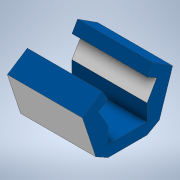
# Autodesk Inventor part: защёлка_выдача
Saved by Autodesk Inventor 2020 (Build 240168000, 168)
## iProperties
Created: 2022-07-29
Part Number: защёлка_выдача
Material: Типовые
Document SubType Name: Modeling
Designer: akapu
Density: 1 g/cm^3
Appearance: По умолчанию
Author: akapu
Autodesk Inventor part; units mm, degrees
ref_plane "YZ Plane" through (0, 0, 0) normal (1, 0, 0) x (0, 1, 0)
ref_plane "XZ Plane" through (0, 0, 0) normal (0, 1, 0) x (-1, 0, 0)
ref_plane "XY Plane" through (0, 0, 0) normal (0, 0, 1) x (1, 0, 0)
sketch "Эскиз8" plane through (0, 0, 0) normal (1, 0, 0) x (0, 1, 0)
  line L0 (0, 0) -> (10.4, 0)
  line L1 (10.4, 0) -> (10.4, -10.4)
  line L2 (10.4, -10.4) -> (0, -10.4)
  line L3 (0, -10.4) -> (0, 0)
  line L4 (5.2, 0) -> (5.2, 4)
  line L5 (5.2, -10.4) -> (5.2, -14.4)
  circle A0 centre (5.2, 4) radius 1.6
  circle A1 centre (5.2, -14.4) radius 1.6
  line L6 (5.2, 4) -> (7.9, 4)
  line L7 (7.9, 2.4412) -> (5.2, 0.8823)
  line L8 (5.2, 0.8823) -> (2.5, 2.4412)
  line L9 (2.5, 2.4412) -> (2.5, 5.5588)
  line L10 (2.5, 5.5588) -> (5.2, 7.1177)
  line L11 (5.2, 7.1177) -> (7.9, 5.5588)
  line L12 (7.9, 5.5588) -> (7.9, 2.4412)
  line L13 (7.9, -15.9588) -> (5.2, -17.5177)
  line L14 (5.2, -17.5177) -> (2.5, -15.9588)
  line L15 (2.5, -15.9588) -> (2.5, -12.8412)
  line L16 (2.5, -12.8412) -> (5.2, -11.2823)
  line L17 (5.2, -11.2823) -> (7.9, -12.8412)
  line L18 (7.9, -12.8412) -> (7.9, -15.9588)
  circle A2 centre (5.2, 4) radius 5.2
  circle A3 centre (5.2, -14.4) radius 5.2
  line L19 (10.4, 4) -> (10.4, 0)
  line L20 (10.4, -10.4) -> (10.4, -14.4)
  line L21 (0, -14.4) -> (0, -10.4)
  line L22 (0, 4) -> (0, 0)
  line L23 (7.9, 5.5588) -> (7.9, 8.4441)
  line L24 (2.5, 5.5588) -> (2.5, 8.4441)
  line L25 (2.5, -15.9588) -> (2.5, -18.8441)
  line L26 (7.9, -15.9588) -> (7.9, -18.8441)
  line L27 (0, 0) -> (-3, 0)
  line L28 (-3, 0) -> (-3, -10.4)
  line L29 (-3, -10.4) -> (0, -10.4)
  line L30 (0, -10.4) -> (0, 0)
  line L31 (10.4, 0) -> (8.9, 2.5981)
  line L32 (10.4, -10.4) -> (8.9, -12.9981)
  line L33 (10.4, -10.4) -> (13.4, -10.4) construction
  line L34 (8.9, -12.9981) -> (4.4, -10.4)
  line L35 (8.9, 2.5981) -> (4.4, 0)
  line L36 (-3, 0) -> (0.663, 6.5408)
  line L37 (-3, -10.4) -> (0.663, -16.9408)
  line L38 (10.4, 0) -> (12.9981, 1.5)
  line L39 (12.9981, 1.5) -> (9.5707, 6.8173)
  line L40 (10.4, -10.4) -> (12.9981, -11.9)
  line L41 (12.9981, -11.9) -> (9.5707, -17.2173)
  point P0 (7.9, -14.4)
  dimension "d51" = 10.4
  dimension "d52" = 10.4
  dimension "d53" = 4
  dimension "d54" = 4
  dimension "d55" = 3.2
  dimension "d56" = 3.2
  dimension "d57" = 2.7
  dimension "d58" = 3
  dimension "d59" = 3
  dimension "d60" = 3
  dimension "d61" = 120
  dimension "d62" = 3
  dimension "d63" = 3
  constraints: 84 end point, 12 point on circle, 7 tangent, 6 coincident, 6 parallel, 6 point on line, 5 perpendicular, 4 centre point, 4 midpoint, 4 vertical, 3 horizontal, 1 collinear, 1 equal length, 26 other
  measures "d51" distance of L1.end L2.end
  measures "d52" distance of L0.end L1.end
  measures "d53" distance of L4.start L4.end
  measures "d54" distance of L5.start L5.end
  measures "d55" diameter of A0
  measures "d56" diameter of A1
  measures "d57" distance of L6.start L6.end
  measures "d58" distance of L29.end L28.end
  measures "d59" distance of L0.end L31.end
  measures "d60" distance of L1.end L32.end
  measures "d61" angle of L32 L33
  measures "d62" distance of L0.end L38.end
  measures "d63" distance of L1.end L40.end
extrude "Выдавливание6" add sketch "Эскиз8" along normal blind 5 contours L0 A2 L24 L9 L8 L4 L35 | L0 L22 A2 | L4 L7 L12 L23 A2 L31 L35 | L27 L36 A2 L22 | L3 L29 L28 L27 | L31 A2 L19 | L19 A2 L39 L38 | L2 A3 L21 | L21 A3 L37 L29 | L40 L41 A3 L20 | L20 A3 L32 | L2 L34 L5 L16 L15 L25 A3 | A3 L26 L18 L17 L5 L34 L32
sketch "Эскиз9" plane through (0, 0, 0) normal (-1, 0, 0) x (0, 0, 1)
  arc A0 (-18.8441, 2.5) -> (-16.9408, 0.663) centre (-14.4, 5.2) ccw projected
  circle A1 centre (-14.4, 5.2) radius 5.2
  circle A2 centre (-14.4, 5.2) radius 1.6
  arc A3 (6.5408, 0.663) -> (8.4441, 2.5) centre (4, 5.2) ccw projected
  circle A4 centre (4, 5.2) radius 5.2
  circle A5 centre (4, 5.2) radius 1.6
  line L0 (2.5981, 8.9) -> (0, 10.4) projected
  line L1 (0, 10.4) -> (2.5981, 8.9)
  line L2 (0, 4.4) -> (2.5981, 8.9) projected
  line L3 (2.5981, 8.9) -> (0, 4.4)
  line L4 (0, 0) -> (0, 4.4) projected
  line L5 (0, 4.4) -> (0, 0)
  line L6 (-10.4, 4.4) -> (-10.4, 0) projected
  line L7 (0, 0) -> (-10.4, 0)
  line L8 (-10.4, 0) -> (-10.4, 1.8774)
  line L9 (-10.4, 10.4) -> (-12.9981, 8.9) projected
  line L10 (-11.699, 9.65) -> (-10.4, 10.4)
  line L11 (-11.9, 12.9981) -> (-10.4, 10.4) projected
  line L12 (-10.4, 10.4) -> (-11.9, 12.9981)
  line L13 (-17.2173, 9.5707) -> (-11.9, 12.9981) projected
  line L14 (-11.9, 12.9981) -> (-17.2173, 9.5707)
  line L15 (0, 10.4) -> (1.5, 12.9981) projected
  line L16 (0, 10.4) -> (1.5, 12.9981)
  line L17 (1.5, 12.9981) -> (6.8173, 9.5707) projected
  line L18 (1.5, 12.9981) -> (6.8173, 9.5707)
  line L19 (0, -3) -> (-10.4, -3) projected
  line L20 (0, -3) -> (6.5408, 0.663)
  line L21 (6.5408, 0.663) -> (0, -3) projected
  line L22 (-10.4, -3) -> (-16.9408, 0.663)
  line L23 (-10.4, -3) -> (-16.9408, 0.663) projected
  line L24 (-10.4, -3) -> (0, -3)
  line L25 (-10.4, 0) -> (0, 0) projected
  line L26 (0, 0) -> (-10.4, 0)
  line L27 (-10.4, 0) -> (-10.4, 1.8774)
  line L28 (0, 1.8774) -> (0, 0)
  line L29 (-11.699, 9.65) -> (-12.9981, 8.9)
  line L30 (-12.9981, 8.9) -> (-10.4, 4.4) projected
  line L31 (-10.4, 4.4) -> (-12.9981, 8.9)
  line L32 (-12.9981, 8.9) -> (-10.4, 4.4)
  line L33 (-10.4, 4.4) -> (-10.4, 1.8774)
  line L34 (0, 1.8774) -> (0, 4.4)
  line L35 (2.5981, 8.9) -> (0, 4.4)
  line L36 (1.299, 9.65) -> (2.5981, 8.9)
  point P0 (-18.8441, 2.5)
  point P1 (-16.9408, 0.663)
  point P2 (6.5408, 0.663)
  point P3 (8.4441, 2.5)
  dimension "d66" = 3.2
  dimension "d67" = 3.2
  constraints: 46 end point, 14 collinear, 4 centre point, 4 coincident, 4 perpendicular, 4 point on circle, 3 point on line, 2 horizontal, 2 midpoint, 2 tangent, 1 parallel
  measures "d66" diameter of A2
  measures "d67" diameter of A5
extrude "Выдавливание7" add sketch "Эскиз9" along normal blind 5 contours A1 L9 L30 L6 A0 | A1 L6 L7 L4 A4 L20 L19 L22 | L13 L11 L9 A1 | A4 L4 L2 L0 A3 | L0 L15 L17 A4
sketch "Эскиз10" plane through (5, 0, 0) normal (1, 0, 0) x (0, 0, -1)
  line L0 (-1.5, 12.9981) -> (-6.8173, 9.5707) projected
  line L1 (0, 10.4) -> (-1.5, 12.9981) projected
  line L2 (-1.5, 12.9981) -> (0, 10.4)
  line L3 (-2.5981, 8.9) -> (0, 10.4) projected
  line L4 (0, 10.4) -> (-2.5981, 8.9)
  line L5 (0, 4.4) -> (-2.5981, 8.9) projected
  line L6 (-2.5981, 8.9) -> (0, 4.4)
  line L7 (0, 0) -> (0, 4.4) projected
  line L8 (0, 4.4) -> (0, 0)
  line L9 (10.4, 0) -> (0, 0) projected
  line L10 (0, 0) -> (10.4, 0)
  line L11 (10.4, 4.4) -> (10.4, 0) projected
  line L12 (10.4, 0) -> (10.4, 4.4)
  line L13 (10.4, 10.4) -> (12.9981, 8.9) projected
  line L14 (10.4, 4.4) -> (12.9981, 8.9)
  line L15 (12.9981, 8.9) -> (10.4, 10.4)
  line L16 (11.9, 12.9981) -> (10.4, 10.4) projected
  line L17 (10.4, 10.4) -> (11.9, 12.9981)
  line L18 (17.2173, 9.5707) -> (11.9, 12.9981) projected
  line L19 (11.9, 12.9981) -> (17.2173, 9.5707)
  line L20 (17.2173, 9.5707) -> (13.6704, -1.1685)
  line L21 (10.4, -3) -> (16.9408, 0.663) projected
  line L22 (10.4, -3) -> (13.6704, -1.1685)
  line L23 (0, -3) -> (10.4, -3) projected
  line L24 (-6.5408, 0.663) -> (0, -3) projected
  line L25 (10.4, -3) -> (0, -3)
  arc A0 (-8.4441, 2.5) -> (-6.5408, 0.663) centre (-4, 5.2) ccw projected
  line L26 (0, -3) -> (-6.5408, 0.663)
  line L27 (-3.2704, -1.1685) -> (-6.8173, 9.5707)
  line L28 (-6.8173, 9.5707) -> (-1.5, 12.9981)
  constraints: 32 end point, 9 collinear, 3 perpendicular, 2 midpoint, 1 tangent
extrude "Выдавливание8" add sketch "Эскиз10" along normal blind 157.53
sketch "Эскиз13" plane through (162.53, 0, 0) normal (1, 0, 0) x (0, 0, -1)
  line L0 (-6.8173, 9.5707) -> (-1.5, 12.9981) projected
  line L1 (-1.5, 12.9981) -> (-6.8173, 9.5707)
  line L2 (-6.5408, 0.663) -> (-3.2704, -1.1685) projected
  line L3 (-6.8173, 9.5707) -> (-3.2704, -1.1685)
  line L4 (-3.2704, -1.1685) -> (0, -3)
  line L5 (10.4, -3) -> (0, -3) projected
  line L6 (0, -3) -> (10.4, -3)
  line L7 (16.9408, 0.663) -> (10.4, -3) projected
  line L8 (10.4, -3) -> (13.6704, -1.1685)
  line L9 (13.6704, -1.1685) -> (17.2173, 9.5707) projected
  line L10 (17.2173, 9.5707) -> (13.6704, -1.1685)
  arc A0 (16.9408, 0.663) -> (17.2173, 9.5707) centre (14.4, 5.2) ccw projected
  line L11 (17.2173, 9.5707) -> (11.9, 12.9981) projected
  line L12 (17.2173, 9.5707) -> (11.9, 12.9981)
  line L13 (11.9, 12.9981) -> (10.4, 10.4) projected
  line L14 (11.9, 12.9981) -> (10.4, 10.4)
  line L15 (10.4, 10.4) -> (12.9981, 8.9) projected
  line L16 (10.4, 10.4) -> (12.9981, 8.9)
  line L17 (12.9981, 8.9) -> (10.4, 4.4)
  line L18 (10.4, 4.4) -> (12.9981, 8.9) projected
  line L19 (0, 0) -> (10.4, 0) projected
  line L20 (10.4, 4.4) -> (10.4, 0)
  line L21 (10.4, 0) -> (0, 0)
  line L22 (0, 4.4) -> (0, 0) projected
  line L23 (0, 0) -> (0, 4.4)
  line L24 (0, 10.4) -> (-2.5981, 8.9) projected
  line L25 (0, 4.4) -> (-2.5981, 8.9)
  line L26 (-2.5981, 8.9) -> (0, 10.4)
  line L27 (-1.5, 12.9981) -> (0, 10.4) projected
  line L28 (0, 10.4) -> (-1.5, 12.9981)
  line L29 (-1.5, 12.9981) -> (11.9, 12.9981)
  line L30 (11.9, 12.9981) -> (11.9, 16.9981)
  line L31 (-1.5, 16.9981) -> (-1.5, 12.9981)
  line L32 (-1.5, 16.9981) -> (0, 16.9981)
  line L33 (0, 20.9981) -> (0, 22.9981)
  line L34 (-1, 23.9981) -> (-0.6923, 23.9981)
  line L35 (-1.5, 21.2778) -> (-1.5, 16.9981)
  line L36 (11.9, 16.9981) -> (10.4, 16.9981)
  line L37 (10.4, 20.9981) -> (10.4, 22.9981)
  line L38 (11.4, 23.9981) -> (11.0923, 23.9981)
  line L39 (11.9, 21.2778) -> (11.9, 16.9981)
  line L40 (-1.5, 23.9981) -> (-1.5, 22.4981)
  line L41 (-6.8173, 9.5707) -> (-3.2704, -1.1685) projected
  arc A1 (-2.3689, 21.6153) -> (-6.8173, 9.5707) centre (10.1732, 10.1395) ccw
  arc A2 (17.2173, 9.5707) -> (12.7689, 21.6153) centre (0.2268, 10.1395) ccw
  line L42 (11.9, 12.9981) -> (19.7387, 7.9454)
  line L43 (-1.5, 12.9981) -> (-9.3387, 7.9454)
  arc A3 (-2.1057, 23.413) -> (-9.3387, 7.9454) centre (15.5626, 5.726) ccw
  arc A4 (19.7387, 7.9454) -> (12.5057, 23.413) centre (-5.1626, 5.726) ccw
  line L44 (13.6704, -1.1685) -> (16.2685, -2.6685)
  line L45 (13.6704, -1.1685) -> (16.6704, -1.1685) construction
  line L46 (-3.2704, -1.1685) -> (-5.8685, -2.6685)
  line L47 (-3.2704, -1.1685) -> (-0.2704, -1.1685) construction
  line L48 (0, -3) -> (-6.5408, 0.663) projected
  line L49 (0, -3) -> (-3.7158, -6.3971)
  line L50 (10.4, -3) -> (14.1158, -6.3971)
  spline S0 degree 2 poles (-1.6495, -2.0762) (-2.6908, -8.8998) (-6.9021, -5.2438) knots 0 0 0 1 1 1
  spline S1 degree 2 poles (12.0352, -2.0842) (13.0969, -8.8932) (17.2999, -5.2483) knots 0 0 0 1 1 1
  arc A5 (-9.3387, 7.9454) -> (-6.9021, -5.2438) centre (15.5626, 5.726) ccw
  arc A6 (17.2999, -5.2483) -> (19.7387, 7.9454) centre (-5.1626, 5.726) ccw
  arc A7 (12.7689, 21.6153) -> (11.9, 21.2778) centre (12.4, 21.2778) ccw
  arc A8 (-1.5, 21.2778) -> (-2.3689, 21.6153) centre (-2, 21.2778) ccw
  arc A9 (-0.6923, 23.9981) -> (-2.1057, 23.413) centre (-0.6923, 21.9981) ccw
  arc A10 (12.5057, 23.413) -> (11.0923, 23.9981) centre (11.0923, 21.9981) ccw
  arc A11 (11.4, 23.9981) -> (10.4, 22.9981) centre (11.4, 22.9981) ccw
  arc A12 (0, 22.9981) -> (-1, 23.9981) centre (-1, 22.9981) ccw
  line L51 (1, 19.9981) -> (9.4, 19.9981)
  line L52 (10.4, 16.9981) -> (9.687, 16.9981)
  line L53 (9.687, 16.9981) -> (0, 16.9981)
  arc A13 (0, 20.9981) -> (1, 19.9981) centre (1, 20.9981) ccw
  arc A14 (9.4, 19.9981) -> (10.4, 20.9981) centre (9.4, 20.9981) ccw
  point P0 (0, 23.9981)
  point P1 (10.4, 23.9981)
  point P2 (11.9, 23.9981)
  point P3 (11.9, 22.4981)
  point P4 (0, 19.9981)
  point P5 (10.4, 19.9981)
  point P6 (-6.9021, -5.2438)
  point P7 (-2.7015, -5.4698)
  point P8 (-1.6495, -2.0762)
  point P9 (12.0352, -2.0842)
  point P10 (13.0907, -5.4599)
  point P11 (11.2726, 23.9899)
  point P12 (-0.8726, 23.9899)
  dimension "d78" = 4
  dimension "d80" = 1.5
  dimension "d81" = 1.5
  dimension "d82" = 17
  dimension "d83" = 17
  dimension "d85" = 9.326
  dimension "d86" = 9.326
  dimension "d87" = 25
  dimension "d88" = 25
  dimension "d89" = 3
  dimension "d90" = 30
  dimension "d91" = 3
  dimension "d92" = 150
  dimension "d94" = 0.5
  dimension "d95" = 2
  dimension "d96" = 1
  dimension "d99" = 1
  constraints: 78 end point, 32 point on circle, 19 point on line, 16 tangent, 14 centre point, 10 collinear, 7 perpendicular, 6 horizontal, 5 equal radius, 5 parallel, 2 equal length, 2 midpoint, 6 other
  measures "d78" distance of L30.end L29.end
  measures "d80" distance of point (10.4, 23.998) point (11.9, 23.998)
  measures "d81" distance of L40.start L40.end
  measures "d82" radius of A1
  measures "d83" radius of A2
  measures "d85" distance of L29.end L42.end
  measures "d86" distance of L0.end L43.end
  measures "d87" radius of A3
  measures "d88" radius of A4
  measures "d89" distance of L8.end L44.end
  measures "d90" angle of L44 L45
  measures "d91" distance of L2.end L46.end
  measures "d92" angle of L46 L47
  measures "d94" radius of A7
  measures "d95" radius of A9
  measures "d96" radius of A11
  measures "d99" radius of A13
extrude "Выдавливание10" add sketch "Эскиз13" along normal blind 10 contours L43 A3 A9 A12 L33 A13 L51 A14 L37 A11 A10 A4 L42 A2 A7 L39 L36 L52 L53 L32 L35 A8 A1 | L3 L4 S0 L49 A5 L43 | A0 L7 L9 | L42 A6 S1 L50 L7 A0 | S0 L49 | L50 S1
sketch "Эскиз15" plane through (172.53, 0, 0) normal (1, 0, 0) x (0, 0, -1)
  arc A0 (-8.4441, 2.5) -> (-6.5408, 0.663) centre (-4, 5.2) ccw projected
  arc A1 (-2.1057, 23.413) -> (-6.9021, -5.2438) centre (15.5626, 5.726) ccw projected
  spline S0 degree 2 poles (-1.6495, -2.0762) (-9.2024, -10.4533) (-8.4441, 2.5) knots 0 0 0 1 1 1
  line L0 (10.4, -3) -> (12.0352, -2.0842) projected
  line L1 (18.8441, 2.5) -> (14.882, 2.5) projected
  arc A2 (17.2999, -5.2483) -> (12.5057, 23.413) centre (-5.1626, 5.726) ccw projected
  spline S1 degree 2 poles (12.0352, -2.0842) (19.6046, -10.4586) (18.8441, 2.5) knots 0 0 0 1 1 1
  line L2 (18.6354, -3) -> (19.4948, 1.6016)
  line L3 (-8.235, -3) -> (-9.0948, 1.6016)
  line L4 (-1.6495, -2.0762) -> (-3.2704, -1.1685) projected
  spline S2 degree 2 poles (-1.6495, -2.0762) (-2.6908, -8.8998) (-6.9021, -5.2438) knots 0 0 0 1 1 1
  spline S3 degree 2 poles (12.0352, -2.0842) (13.0969, -8.8932) (17.2999, -5.2483) knots 0 0 0 1 1 1
  point P0 (0, 0)
  point P1 (-3.7158, -6.3971)
  point P2 (14.1158, -6.3971)
  constraints: 4 end point, 2 point on circle, 1 point on line, 15 other
extrude "Выдавливание11" cut sketch "Эскиз15" against normal blind 10
sketch "Эскиз16" plane through (172.53, 0, 0) normal (1, 0, 0) x (0, 0, -1)
  line L0 (-1.6495, -2.0762) -> (-3.2704, -1.1685) projected
  line L1 (-2.4412, 2.5) -> (-8.4441, 2.5) projected
  arc A0 (-2.1057, 23.413) -> (-6.9021, -5.2438) centre (15.5626, 5.726) ccw projected
  spline S0 degree 2 poles (-1.6495, -2.0762) (-9.2024, -10.4533) (-8.4441, 2.5) knots 0 0 0 1 1 1
  line L2 (13.6704, -1.1685) -> (12.0352, -2.0842) projected
  arc A1 (16.9408, 0.663) -> (18.8441, 2.5) centre (14.4, 5.2) ccw projected
  arc A2 (17.2999, -5.2483) -> (12.5057, 23.413) centre (-5.1626, 5.726) ccw projected
  spline S1 degree 2 poles (12.0352, -2.0842) (19.6046, -10.4586) (18.8441, 2.5) knots 0 0 0 1 1 1
  line L3 (-1.6495, -2.0762) -> (0, -3) projected
  line L4 (-1.6495, -2.0762) -> (-8.4702, -1.1606)
  line L5 (12.0352, -2.0842) -> (18.8706, -1.1592)
  line L6 (-8.235, -3) -> (-9.0071, 1.1077)
  line L7 (18.6354, -3) -> (19.4075, 1.1099)
  point P0 (0, 0)
  point P1 (18.7195, -2.5523)
  point P2 (-8.319, -2.5532)
  constraints: 8 end point, 4 point on circle, 2 tangent, 10 other
extrude "Выдавливание12" add sketch "Эскиз16" against normal blind 10
sketch "Эскиз17" plane through (-5, 0, 0) normal (-1, 0, 0) x (0, 0, 1)
  line L0 (-37.7292, 41.1824) -> (41.3103, 41.1824)
  line L1 (41.3103, 41.1824) -> (41.3103, -34.7876)
  line L2 (41.3103, -34.7876) -> (-37.7292, -34.7876)
  line L3 (-37.7292, -34.7876) -> (-37.7292, 41.1824)
  point P0 (0, 0)
  constraints: 8 end point, 2 parallel, 1 horizontal, 1 perpendicular
extrude "Выдавливание13" cut sketch "Эскиз17" against normal blind 147.53
sketch "Эскиз18" plane through (172.53, 0, 0) normal (1, 0, 0) x (0, 0, -1)
  line L0 (-31.4647, -11.5956) -> (67.799, -11.5956)
  line L1 (67.799, -11.5956) -> (67.799, 38.6102)
  line L2 (67.799, 38.6102) -> (-31.4647, 38.6102)
  line L3 (-31.4647, 38.6102) -> (-31.4647, -11.5956)
  point P0 (0, 0)
  constraints: 8 end point, 2 parallel, 1 horizontal, 1 perpendicular
extrude "Выдавливание14" cut sketch "Эскиз18" against normal blind 10
